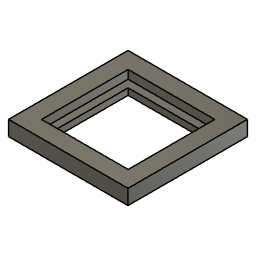
Switch Tolerance Test (14.4mm, 1.3mm) (Autodesk Fusion 360 design; units mm, degrees)
Autodesk Fusion 360 part; units mm, degrees
sketch "Sketch1" plane through (0, 0, 0) normal (0, 1, 0) x (1, 0, 0)
  line L0 (-7.1721, 7.2) -> (7.2279, 7.2)
  line L1 (-8.6721, -8.7) -> (-8.6721, 8.7)
  line L2 (7.2279, -7.2) -> (-7.1721, -7.2)
  line L3 (-8.6721, 8.7) -> (8.7279, 8.7)
  line L4 (-8.6721, -8.7) -> (8.7279, 8.7) construction
  line L5 (-7.1721, -7.2) -> (7.2279, 7.2) construction
  line L6 (8.7279, -8.7) -> (-8.6721, -8.7)
  line L7 (-7.1721, -7.2) -> (-7.1721, 7.2)
  line L8 (7.2279, 7.2) -> (7.2279, -7.2)
  line L9 (8.7279, 8.7) -> (8.7279, -8.7)
  line L10 (8.7279, -8.7) -> (-8.6721, 8.7) construction
  line L11 (7.2279, -7.2) -> (-7.1721, 7.2) construction
  line L12 (-12, 12) -> (12, 12)
  line L13 (12, 12) -> (12, -12)
  line L14 (12, -12) -> (-12, -12)
  line L15 (-12, -12) -> (-12, 12)
  line L16 (-12, 12) -> (12, -12) construction
  line L17 (12, 12) -> (-12, -12) construction
  point P0 (0.0279, 0)
  dimension "d1" = 14.4
  dimension "d2" = 14.4
  dimension "d3" = 1.5
  dimension "d4" = 1.5
  dimension "d5" = 1.5
  dimension "d6" = 1.5
  dimension "d7" = 24
  dimension "d8" = 24
  constraint horizontal L2
  constraint perpendicular L2 L7
  constraint parallel L0 L2
  constraint parallel L7 L8
  constraint coincident P0 L11
  constraint coincident P0 L5
  constraint horizontal L6
  constraint perpendicular L1 L6
  constraint parallel L3 L6
  constraint parallel L1 L9
  constraint horizontal origin P0
  constraint horizontal L12
  constraint perpendicular L12 L13
  constraint parallel L12 L14
  constraint parallel L13 L15
  constraint coincident L16 origin
  constraint coincident L17 origin
  measures "d1" distance of L0.end L0.start
  measures "d2" distance of L2.end L0.start
  measures "d3" distance of L2 L6
  measures "d4" distance of L8 L9
  measures "d5" distance of L0 L3
  measures "d6" distance of L1 L7
  measures "d7" distance of L13.end L14.end
  measures "d8" distance of L12.end L13.end
extrude "Extrude1" add sketch "Sketch1" along normal blind 3 contours L12 L13 L14 L15
extrude "Extrude2" add sketch "Sketch1" along normal blind 1.3 contours L1 L3 L6 L9
